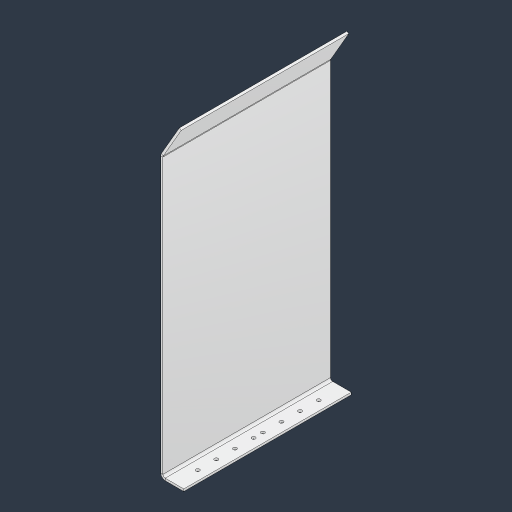
# Autodesk Inventor part: trough_back_support
Saved by Autodesk Inventor 2024.3 (Build 283343000, 343)
## iProperties
Created: 2025-03-03
Part Number: trough_back_support
Material: Aluminum 6061
Document SubType Name: Sheet Metal
Designer: marcu
Mass: 862.25 g
Surface Area: 2141.31 cm^2
Volume: 319.352 cm^3
Density: 2.7 g/cm^3
Sheet Metal Rule: Default
Appearance: Aluminum - Flat
Author: marcu
Autodesk Inventor part; units mm, degrees
ref_plane "YZ Plane" through (0, 0, 0) normal (1, 0, 0) x (0, 1, 0)
ref_plane "XZ Plane" through (0, 0, 0) normal (0, 1, 0) x (-1, 0, 0)
ref_plane "XY Plane" through (0, 0, 0) normal (0, 0, 1) x (1, 0, 0)
sketch "Sketch1" plane through (0, 0, 0) normal (0, 1, 0) x (-1, 0, 0)
  line L0 (-12.7, -114.3) -> (12.7, -114.3)
  line L1 (12.7, -114.3) -> (12.7, 114.3)
  line L2 (12.7, 114.3) -> (-12.7, 114.3)
  line L3 (-12.7, 114.3) -> (-12.7, -114.3)
  line L4 (-12.7, -114.3) -> (12.7, 114.3) construction
  line L5 (12.7, -114.3) -> (-12.7, 114.3) construction
  point P0 (0, 0)
  dimension "d0" = 25.4
  dimension "d1" = 228.6
  measures "d0" distance of L2.end L1.end
  measures "d1" distance of L0.end L1.end
extrude "Plate1" add sketch "Sketch1" along normal blind 3.048
sketch "Sketch2" plane through (-15.748, 6.096, 114.3) normal (-1, 0, 0) x (0, -1, 0)
  line L0 (0, -228.6) -> (0, 0)
  line L1 (0, 0) -> (-374.904, 0)
  line L2 (-374.904, 0) -> (-374.904, -228.6)
  line L3 (-374.904, -228.6) -> (0, -228.6)
  constraints: 6 end point, 1 horizontal, 1 perpendicular, 1 vertical
edge flange "Flange1" height 381 angle 90 thickness 3.048 bend radius 3.048 thickness toward (-1, 0, 0) relief straight relief width 3.048 relief depth 1.524 edges at (-12.7, 3.048, 0) wall of the first edge with corners at (-15.748, 6.096, -114.3) (-15.748, 6.096, 114.3) (-15.748, 381, 114.3) (-15.748, 381, -114.3)
bend "Bend1"
corner "Corner1"
sketch "Sketch3" plane through (0, 3.048, 0) normal (0, 1, 0) x (1, 0, 0)
  line L0 (-12.7, 114.3) -> (12.7, 114.3) construction
  line L1 (-12.7, -114.3) -> (-12.7, 114.3) construction
  line L2 (12.7, -114.3) -> (-12.7, -114.3) construction
  line L3 (12.7, 114.3) -> (12.7, -114.3) construction
  line L4 (12.7, 0) -> (-12.7, 0) construction
  point P0 (0, 0)
  point P1 (0, -6.35)
  point P2 (0, 0)
  point P3 (0, -31.75)
  point P4 (0, -57.15)
  point P5 (0, -82.55)
  point P6 (0, -107.95)
  point P7 (0, 6.35)
  point P8 (0, 31.75)
  point P9 (0, 57.15)
  point P10 (0, 82.55)
  point P11 (0, 107.95)
  dimension "d13" = 6.35
  dimension "d16" = 25.4
  dimension "d21" = 12.7
  constraints: 5 symmetric about line, 3 midpoint, 2 end point, 1 vertical, 4 other
  measures "d13" distance of point (0, 0) point (0, -6.35)
  measures "d16" distance of point (0, -6.35) point (0, -31.75)
  measures "d21" distance from line of L3 point (0, -6.35)
hole "Hole1" at (0, 3.048, 6.35) at (0, 3.048, 31.75) at (0, 3.048, 57.15) at (0, 3.048, 82.55) at (0, 3.048, -82.55) at (0, 3.048, -57.15) at (0, 3.048, -31.75) at (0, 3.048, -6.35) direction (0, -1, 0) diameter 5.1054 end through all clearance for "Flat Head Machine Screw (82)" size "#10" standard "Ansi Unified Screw Threads"
sketch "Sketch4" plane through (-15.3396, 382.524, 114.3) normal (-0.8660254, 0.5, 0) x (-0.5, -0.8660254, 0)
  line L0 (0, -228.6) -> (0, 0)
  line L1 (0, 0) -> (-49.1666, 0)
  line L2 (-49.1666, 0) -> (-49.1666, -228.6)
  line L3 (-49.1666, -228.6) -> (0, -228.6)
  constraints: 6 end point, 1 horizontal, 1 perpendicular, 1 vertical
edge flange "Flange2" height 50.8 angle 30 thickness 3.048 bend radius 3.048 thickness toward (-0.8660254, 0.5, 0) relief straight relief width 3.048 relief depth 1.524 edges at (-15.748, 381, 0) wall of the first edge with corners at (-15.3396, 382.524, -114.3) (-15.3396, 382.524, 114.3) (9.2436, 425.1035, 114.3) (9.2436, 425.1035, -114.3)
bend "Bend2"
corner "Corner2"
equation "\"d27\" = Thickness"
equation "\"d2\" = Thickness"
equation "\"d3\" = BendReliefWidth"
equation "\"d4\" = BendReliefDepth"
equation "\"d5\" = MinimumRemnant"
equation "\"d6\" = TransitionRadius"
equation "\"d9\" = BendRadius"
equation "\"d10\" = CornerReliefSize"
equation "\"d11\" = GapSize"
equation "\"d12\" = JacobiRadiusSize"
equation "\"d29\" = BendReliefWidth"
equation "\"d30\" = BendReliefDepth"
equation "\"d31\" = MinimumRemnant"
equation "\"d32\" = TransitionRadius"
equation "\"d35\" = BendRadius"
equation "\"d36\" = CornerReliefSize"
equation "\"d37\" = GapSize"
equation "\"d38\" = JacobiRadiusSize"
equation "\"BendRadius\" = Thickness"
equation "\"BendReliefWidth\" = Thickness"
equation "\"BendReliefDepth\" = 0.5 * Thickness"
equation "\"CornerReliefSize\" = 4 * Thickness"
equation "\"MinimumRemnant\" = 2 * Thickness"
equation "\"TransitionRadius\" = BendRadius"
equation "\"JacobiRadiusSize\" = BendRadius"
equation "\"GapSize\" = Thickness"
equation "\"Thickness\" = 3.048"
body "Solid1"
